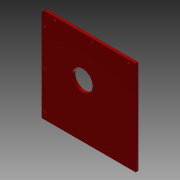
# Autodesk Inventor part: Module Plate - Bottom
Saved by Autodesk Inventor 2013 (Build 170138000, 138)
## iProperties
Created: 2013-04-01
Part Number: Module Plate - Bottom
Material: Generic
Document SubType Name: Modeling
Designer: mvarma
Density: 1 g/cm^3
Author: mvarma
Autodesk Inventor part; units mm, degrees
ref_plane "YZ Plane" through (0, 0, 0) normal (1, 0, 0) x (0, 1, 0)
ref_plane "XZ Plane" through (0, 0, 0) normal (0, 1, 0) x (-1, 0, 0)
ref_plane "XY Plane" through (0, 0, 0) normal (0, 0, 1) x (1, 0, 0)
sketch "Sketch1" plane through (0, 0, 0) normal (0, 0, 1) x (1, 0, 0)
  line L0 (0, 0) -> (152.4, 0)
  line L1 (152.4, 0) -> (152.4, -152.4)
  line L2 (152.4, -152.4) -> (0, -152.4)
  line L3 (0, -152.4) -> (0, 0)
  line L4 (0, -152.4) -> (-50.8, -152.4) construction
  line L5 (-50.8, -152.4) -> (-50.8, 25.4) construction
  line L6 (0, 0) -> (0, -152.4)
  line L7 (-47.625, 25.4) -> (152.4, 25.4) construction
  line L8 (152.4, 25.4) -> (152.4, 0) construction
  line L9 (152.4, 0) -> (0, 0)
  line L10 (-47.625, 0) -> (-47.625, 25.4) construction
  line L11 (-50.8, -152.4) -> (-50.8, 25.4) construction
  line L12 (-50.8, 25.4) -> (-47.625, 25.4) construction
  circle A0 centre (60.96, -60.96) radius 54.61 construction
  circle A1 centre (60.96, -60.96) radius 53.34 construction
  circle A2 centre (60.96, -60.96) radius 17.4625
  line L13 (0, 0) -> (-47.625, 0) construction
  line L14 (0, -152.4) -> (-9.525, -152.4)
  line L15 (-9.525, -152.4) -> (-9.525, 3.175)
  line L16 (-3.175, 9.525) -> (152.4, 9.525)
  line L17 (152.4, 0) -> (152.4, 9.525)
  circle A3 centre (60.96, -60.96) radius 47.2059 construction
  line L18 (-4.7625, 9.525) -> (-4.7625, -152.4) construction
  line L19 (-9.525, 4.7625) -> (152.4, 4.7625) construction
  arc A4 (-3.175, 9.525) -> (-9.525, 3.175) centre (-3.175, 3.175) ccw
  point P0 (-9.525, 9.525)
  point P1 (12.7, 4.7625)
  point P2 (-4.7625, -12.7)
  point P3 (76.2, 4.7625)
  point P4 (139.7, 4.7625)
  point P5 (-4.7625, -76.2)
  point P6 (-4.7625, -139.7)
  dimension "d0" = 152.4
  dimension "d8" = 50.8
  dimension "d12" = 3.175
  dimension "d28" = 152.4
  dimension "d29" = 109.22
  dimension "d30" = 106.68
  dimension "d31" = 60.96
  dimension "d32" = 60.96
  dimension "d33" = 34.925
  dimension "d34" = 9.525
  dimension "d35" = 9.525
  dimension "d41" = 94.4118
  dimension "d42" = 25.4
  dimension "d43" = 22.225
  dimension "d44" = 22.225
  dimension "d45" = 6.35
  dimension "d48" = 63.5
  dimension "d55" = 63.5
  constraints: 40 end point, 8 point on line, 7 parallel, 6 perpendicular, 5 centre point, 5 horizontal, 3 coincident, 2 midpoint, 2 point on circle, 2 tangent, 2 vertical, 1 collinear, 4 other
  measures "d0" distance of L0.start L0.end
  measures "d8" distance between parallel lines of L3 L5
  measures "d12" distance between parallel lines of L11 L10
  measures "d28" distance between parallel lines of L4 L9
  measures "d29" diameter of A0
  measures "d30" diameter of A1
  measures "d31" distance from line of L6 A0.centre
  measures "d32" distance from line of L0 A0.centre
  measures "d33" diameter of A2
  measures "d34" distance between parallel lines of L16 L9
  measures "d35" distance between parallel lines of L6 L15
  measures "d41" diameter of A3
  measures "d42" distance between parallel lines of L0 L7
  measures "d43" distance from line of L16 point (-4.762, -12.7)
  measures "d44" distance from line of L15 point (12.7, 4.763)
  measures "d45" radius of A4
  measures "d48" distance of point (12.7, 4.763) point (76.2, 4.763)
  measures "d55" distance of point (-4.762, -12.7) point (-4.762, -76.2)
extrude "Extrusion1" add sketch "Sketch1" along normal blind 4.7625
hole "Hole1" at (12.7, 4.7625, 0) at (-4.7625, -12.7, 0) at (76.2, 4.7625, 0) at (139.7, 4.7625, 0) at (-4.7625, -76.2, 0) at (-4.7625, -139.7, 0) direction (0, 0, 1) diameter 4.9784 end through all clearance for "Socket Head Cap Screw" size "#10" standard "Ansi Unified Screw Threads"
body "Solid1"
